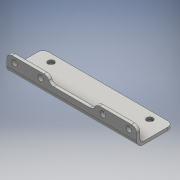
# Autodesk Inventor part: ОПОРА_05
Saved by Autodesk Inventor 2016 (Build 200138000, 138)
## iProperties
Created: 2021-05-03
Part Number: ОПОРА_05
Material: Типовые
Document SubType Name: Modeling
Designer: Лол
Density: 1 g/cm^3
Appearance: По умолчанию
Author: Лол
Autodesk Inventor part; units mm, degrees
ref_plane "YZ Plane" through (0, 0, 0) normal (1, 0, 0) x (0, 1, 0)
ref_plane "XZ Plane" through (0, 0, 0) normal (0, 1, 0) x (-1, 0, 0)
ref_plane "XY Plane" through (0, 0, 0) normal (0, 0, 1) x (1, 0, 0)
sketch "Эскиз1" plane through (0, 0, 0) normal (1, 0, 0) x (0, 1, 0)
  line L0 (-14, 0) -> (84, 0) projected
  line L1 (0, -7) -> (0, 42) projected
  line L2 (0, 35) -> (0, 0)
  line L3 (0, 0) -> (70, 0)
  line L4 (70, 6) -> (6, 6)
  line L5 (6, 6) -> (6, 35)
  line L6 (6, 35) -> (0, 35)
  line L7 (70, 6) -> (70, 0)
  dimension "d50" = 6
  dimension "d51" = 6
  dimension "d52" = 70
  dimension "d53" = 35
  constraints: 12 end point, 3 perpendicular, 2 point on line, 1 collinear, 1 horizontal
  measures "d50" distance between parallel lines of L3 L4
  measures "d51" distance between parallel lines of L2 L5
  measures "d52" distance between parallel lines of L1 L7
  measures "d53" distance between parallel lines of L0 L6
extrude "Выдавливание1" add sketch "Эскиз1" against normal blind 250
fillet "Сопряжение2" radius 6 1 edges at (-125, 6, 6)
fillet "Сопряжение3" radius 12 1 edges at (-125, 0, 0)
sketch "Эскиз5" plane through (-250, 0, 35) normal (0, -1, 0) x (1, 0, 0)
  line L0 (250, 0) -> (250, -23) construction
  line L1 (0, -23) -> (0, 0) construction
  line L2 (250, 0) -> (0, 0) construction
  line L3 (0, -10) -> (250, -10) construction
  circle A0 centre (15, -10) radius 5.25
  circle A1 centre (65, -10) radius 5.25
  circle A2 centre (235, -10) radius 5.25
  circle A3 centre (185, -10) radius 5.25
  point P0 (250, -35)
  dimension "d56" = 10
  dimension "d57" = 15
  dimension "d58" = 50
  dimension "d59" = 220
  dimension "d60" = 50
  dimension "d61" = 10.5
  constraints: 6 point on line, 4 centre point, 3 equal radius, 2 end point, 1 perpendicular
  measures "d56" distance between parallel lines of L3 L2
  measures "d57" distance from line of A0.centre L1
  measures "d58" distance of A1.centre A0.centre
  measures "d59" distance of A2.centre A0.centre
  measures "d60" distance of A3.centre A2.centre
  measures "d61" diameter of A0
extrude "Выдавливание3" cut sketch "Эскиз5" against normal blind 10
fillet "Сопряжение4" radius 10 2 edges at (0, 3, 35) (-250, 3, 35)
sketch "Эскиз6" plane through (-250, 0, 12) normal (0, -1, 0) x (1, 0, 0)
  circle A0 centre (65, 13) radius 5.25 construction
  circle A1 centre (185, 13) radius 5.25 construction
  line L0 (240, 23) -> (10, 23) construction
  line L1 (80, 23) -> (80, 11)
  line L2 (80, 11) -> (170, 11)
  line L3 (170, 11) -> (170, 23)
  line L4 (80, 23) -> (170, 23)
  point P0 (250, -12)
  dimension "d65" = 15
  dimension "d66" = 15
  dimension "d67" = 12
  constraints: 8 end point, 3 perpendicular, 2 point on line, 1 collinear
  measures "d65" distance from line of L1 A0.centre
  measures "d66" distance from line of A1.centre L3
  measures "d67" distance between parallel lines of L2 L0
extrude "Выдавливание4" cut sketch "Эскиз6" against normal blind 10
fillet "Сопряжение5" radius 10 4 edges at (-170, 3, 23) (-80, 3, 23) (-170, 3, 35) (-80, 3, 35)
fillet "Сопряжение6" radius 10 2 edges at (0, 70, 3) (-250, 70, 3)
sketch "Эскиз7" plane through (-250, 12, 6) normal (0, 0, 1) x (1, 0, 0)
  line L0 (240, -12) -> (178.3303, -12) construction
  circle A0 centre (220, 43) radius 6
  circle A1 centre (30, 43) radius 6
  line L1 (250, 48) -> (250, 0) construction
  line L2 (0, 0) -> (0, 48) construction
  point P0 (250, -12)
  dimension "d72" = 55
  dimension "d73" = 12
  dimension "d74" = 30
  dimension "d75" = 30
  dimension "d76" = 55
  constraints: 2 centre point, 1 equal radius
  measures "d72" distance from line of A0.centre L0
  measures "d73" diameter of A0
  measures "d74" distance from line of L1 A0.centre
  measures "d75" distance from line of A1.centre L2
  measures "d76" distance from line of A1.centre L0
extrude "Выдавливание5" cut sketch "Эскиз7" against normal blind 10
